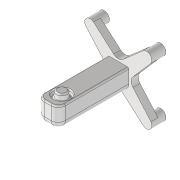
# Autodesk Inventor part: Sensor
Saved by Autodesk Inventor 2020 (Build 240168000, 168)
## iProperties
Created: 2020-03-19
Part Number: Sensor
Material: Generisch
Document SubType Name: Modeling
Designer: franz
Density: 1 g/cm^3
Appearance: Vorgabe
Author: franz
Autodesk Inventor part; units mm, degrees
ref_plane "YZ Plane" through (0, 0, 0) normal (1, 0, 0) x (0, 1, 0)
ref_plane "XZ Plane" through (0, 0, 0) normal (0, 1, 0) x (-1, 0, 0)
ref_plane "XY Plane" through (0, 0, 0) normal (0, 0, 1) x (1, 0, 0)
sketch "Skizze1" plane through (0, 0, 0) normal (0, 0, 1) x (1, 0, 0)
  line L0 (-15, -15) -> (15, -15)
  line L1 (15, -15) -> (15, 15)
  line L2 (15, 15) -> (-15, 15)
  line L3 (-15, 15) -> (-15, -15)
  line L4 (-15, -15) -> (15, 15) construction
  line L5 (15, -15) -> (-15, 15) construction
  point P0 (0, 0)
  dimension "d0" = 30
  dimension "d1" = 30
  constraints: 12 end point, 2 midpoint, 2 parallel, 1 horizontal, 1 perpendicular
  measures "d0" distance of L2.end L1.end
  measures "d1" distance of L1.end L0.end
extrude "Extrusion1" add sketch "Skizze1" along normal blind 100
sketch "Skizze2" plane through (0, 0, 0) normal (0, 0, -1) x (-1, 0, 0)
  circle A0 centre (40, -40) radius 7.5
  circle A1 centre (-40, -40) radius 7.5
  circle A2 centre (-40, 40) radius 7.5
  circle A3 centre (40, 40) radius 7.5
  line L0 (0, -66.5) -> (0, 66.5) projected
  line L1 (66.5, 0) -> (-66.5, 0) projected
  line L2 (45.6471, -35.0643) -> (15, 0)
  line L3 (15, 15) -> (15, -15) projected
  line L4 (35.8038, -46.2162) -> (0, -15)
  line L5 (15, -15) -> (-15, -15) projected
  line L6 (0, -15) -> (-35.0643, -45.6471)
  line L7 (-15, -15) -> (-15, 15) projected
  line L8 (-15, 0) -> (-46.2162, -35.8038)
  line L9 (-15, 15) -> (15, 15) projected
  line L10 (0, 15) -> (-34.4135, 45.0041)
  line L11 (-15, 0) -> (-45.6471, 35.0643)
  line L12 (0, 15) -> (35.0643, 45.6471)
  line L13 (15, 0) -> (45.0041, 34.4135)
  point P0 (0, 0)
  dimension "d4" = 15
  dimension "d5" = 15
  dimension "d6" = 15
  dimension "d7" = 15
  dimension "d8" = 40
  dimension "d9" = 40
  constraints: 16 end point, 8 point on circle, 5 perpendicular, 4 centre point, 4 midpoint, 3 symmetric about line, 2 point on line, 2 tangent
  measures "d4" diameter of A0
  measures "d5" diameter of A1
  measures "d6" diameter of A3
  measures "d7" diameter of A2
  measures "d8" distance from line of A0.centre L1
  measures "d9" distance from line of L0 A0.centre
extrude "Extrusion2" add sketch "Skizze2" along normal blind 10 contours A0 L4 | A0 L4 L5 L3 L2 | L3 L5 L0 L1 | L1 L0 L9 L3 | L3 L9 L12 A3 L13 | L5 L7 L1 L0 | L6 A1 L8 L7 L5 | L1 L7 L9 L0 | A3 | A1 L8 | L9 L7 L11 A2 L10 | A2 picked at (40.9311, -37.6896) picked at (-39.2767, -42.7034)
sketch "Skizze3" plane through (0, 0, -10) normal (0, 0, -1) x (-1, 0, 0)
  arc A0 (45.0041, 34.4135) -> (35.0643, 45.6471) centre (40, 40) ccw projected
  circle A1 centre (40, 40) radius 7.5
  arc A2 (35.8038, -46.2162) -> (45.6471, -35.0643) centre (40, -40) ccw projected
  circle A3 centre (40, -40) radius 7.5
  arc A4 (-46.2162, -35.8038) -> (-35.0643, -45.6471) centre (-40, -40) ccw projected
  circle A5 centre (-40, -40) radius 7.5
  arc A6 (-34.4135, 45.0041) -> (-45.6471, 35.0643) centre (-40, 40) ccw projected
  circle A7 centre (-40, 40) radius 7.5
  point P0 (0, 0)
  point P1 (-45.6471, 35.0643)
  point P2 (-34.4135, 45.0041)
  point P3 (45.6471, -35.0643)
  point P4 (-35.0643, -45.6471)
  point P5 (-46.2162, -35.8038)
  point P6 (35.0643, 45.6471)
  constraints: 4 centre point, 4 coincident
extrude "Extrusion3" add sketch "Skizze3" along normal blind 10
sketch "Skizze4" plane through (-15, 15, 100) normal (0, 1, 0) x (1, 0, 0)
  circle A0 centre (15, 20) radius 12.5
  line L0 (30, 0) -> (0, 0) projected
  point P0 (15, 100)
  dimension "d14" = 25
  dimension "d15" = 20
  constraints: 1 centre point
  measures "d14" diameter of A0
  measures "d15" distance from line of L0 A0.centre
extrude "Extrusion4" cut sketch "Skizze4" against normal blind 5
sketch "Skizze5" plane through (0, 10, 80) normal (0, 1, 0) x (1, 0, 0)
  circle A0 centre (0, 0) radius 7.5
  point P0 (0, 80)
  dimension "d18" = 15
  constraints: 1 centre point
  measures "d18" diameter of A0
extrude "Extrusion5" add sketch "Skizze5" along normal blind 10
fillet "Rundung1" radius 10 2 edges at (15, 0, 100) (-15, 0, 100)
fillet "Rundung2" radius 10 5 edges at (12.0711, -15, 97.0711) (0, -15, 100) (-12.0711, -15, 97.0711) (-15, -15, 45) (15, -15, 45)
chamfer "Fase3" distance 2 angle 45 3 edges at (-7.5, 20, 80) (-7.5, 10, 80) (-12.5, 10, 80)
fillet "Rundung3" radius 2 5 edges at (12.0711, 15, 97.0711) (0, 15, 100) (-12.0711, 15, 97.0711) (-15, 15, 45) (15, 15, 45)
fillet "Rundung4" radius 10 4 edges at (0, -15, -5) (15, 0, -5) (-15, 0, -5) (0, 15, -5)
equation "\"d5\" = d4"
equation "\"d6\" = d4"
equation "\"d7\" = d4"
equation "\"d9\" = d8"
